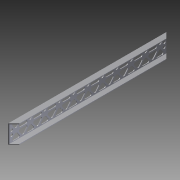
# Autodesk Inventor part: big U channel 3.25in
Saved by Autodesk Inventor 2012 (Build 160160000, 160)
## iProperties
Created: 2013-07-06
Part Number: big U channel 3.25in
Material: Default
Document SubType Name: Modeling
Designer: Bryce
Density: 1 g/cm^3
Author: Bryce
Autodesk Inventor part; units mm, degrees
ref_plane "YZ Plane" through (0, 0, 0) normal (1, 0, 0) x (0, 1, 0)
ref_plane "XZ Plane" through (0, 0, 0) normal (0, 1, 0) x (-1, 0, 0)
ref_plane "XY Plane" through (0, 0, 0) normal (0, 0, 1) x (1, 0, 0)
sketch "Sketch1" plane through (0, 0, 0) normal (0, 0, 1) x (1, 0, 0)
  line L0 (0, 0) -> (25.4, 0)
  line L1 (25.4, 82.55) -> (0, 82.55)
  line L2 (0, 82.55) -> (0, 0)
  line L3 (25.4, 79.375) -> (3.175, 79.375)
  line L4 (3.175, 79.375) -> (3.175, 3.175)
  line L5 (3.175, 3.175) -> (25.4, 3.175)
  line L6 (25.4, 82.55) -> (25.4, 79.375)
  line L7 (25.4, 3.175) -> (25.4, 0)
  dimension "d0" = 82.55
  dimension "d1" = 25.4
  dimension "d2" = 25.4
  dimension "d3" = 3.175
  dimension "d4" = 3.175
  dimension "d5" = 3.175
  constraints: 16 end point, 3 equal length, 3 perpendicular, 2 horizontal
  measures "d0" distance of L1.end L0.start
  measures "d1" distance of L1.start L1.end
  measures "d2" distance of L0.start L0.end
  measures "d3" distance between parallel lines of L1 L3
  measures "d4" distance between parallel lines of L2 L4
  measures "d5" distance between parallel lines of L0 L5
extrude "Extrusion1" add sketch "Sketch1" along normal blind 711.2
sketch "Sketch2" plane through (0, 82.55, 0) normal (0, 1, 0) x (1, 0, 0)
  line L0 (0, -711.2) -> (25.4, -711.2) projected
  line L1 (25.4, 0) -> (25.4, -711.2) projected
  line L2 (25.4, 0) -> (0, 0) projected
  line L3 (0, -711.2) -> (25.4, -685.8)
  line L4 (0, 0) -> (25.4, -25.4)
  dimension "d8" = 45
  constraints: 4 end point, 2 point on line, 1 perpendicular
  measures "d8" angle of L0 L3
extrude "Extrusion2" cut sketch "Sketch2" against normal through all
sketch "Sketch3" plane through (0, 0, 711.2) normal (-1, 0, 0) x (0, 0, 1)
  line L0 (0, 0) -> (0, 82.55) projected
  line L1 (-711.2, 82.55) -> (0, 82.55) projected
  line L2 (-711.2, 82.55) -> (-711.2, 0) projected
  line L3 (-711.2, 0) -> (0, 0) projected
  line L4 (-711.2, 41.275) -> (0, 41.275) construction
  line L5 (-711.2, 0) -> (-646.5455, 82.55) construction
  line L6 (-646.5455, 82.55) -> (-581.8909, 0) construction
  line L7 (-581.8909, 0) -> (-517.2364, 82.55) construction
  line L8 (-517.2364, 82.55) -> (-452.5818, 0) construction
  line L9 (-452.5818, 0) -> (-387.9273, 82.55) construction
  line L10 (-387.9273, 82.55) -> (-323.2727, 0) construction
  line L11 (-323.2727, 0) -> (-258.6182, 82.55) construction
  line L12 (-258.6182, 82.55) -> (-193.9636, 0) construction
  line L13 (-193.9636, 0) -> (-129.3091, 82.55) construction
  line L14 (-129.3091, 82.55) -> (-64.6545, 0) construction
  line L15 (-64.6545, 0) -> (0, 82.55) construction
  line L16 (-711.2, 82.55) -> (-646.5455, 0) construction
  line L17 (-646.5455, 0) -> (-581.8909, 82.55) construction
  line L18 (-581.8909, 82.55) -> (-517.2364, 0) construction
  line L19 (-517.2364, 0) -> (-452.5818, 82.55) construction
  line L20 (-452.5818, 82.55) -> (-387.9273, 0) construction
  line L21 (-387.9273, 0) -> (-323.2727, 82.55) construction
  line L22 (-323.2727, 82.55) -> (-258.6182, 0) construction
  line L23 (-258.6182, 0) -> (-193.9636, 82.55) construction
  line L24 (-193.9636, 82.55) -> (-129.3091, 0) construction
  line L25 (-129.3091, 0) -> (-64.6545, 82.55) construction
  line L26 (-64.6545, 82.55) -> (0, 0) construction
  line L27 (-702.1937, 6.35) -> (-678.8727, 36.1258)
  line L28 (-678.8727, 36.1258) -> (-655.5518, 6.35)
  line L29 (-655.5518, 6.35) -> (-702.1937, 6.35)
  line L30 (-672.3531, 38.1) -> (-646.5455, 5.1492)
  line L31 (-646.5455, 5.1492) -> (-620.7378, 38.1)
  line L32 (-620.7378, 38.1) -> (-672.3531, 38.1)
  line L33 (-704.85, 13.2568) -> (-685.3924, 38.1)
  line L34 (-685.3924, 38.1) -> (-704.85, 38.1)
  line L35 (-704.85, 38.1) -> (-704.85, 13.2568)
  line L36 (-704.85, 69.2932) -> (-704.85, 44.45)
  line L37 (-704.85, 44.45) -> (-685.3924, 44.45)
  line L38 (-685.3924, 44.45) -> (-704.85, 69.2932)
  line L39 (-702.1937, 76.2) -> (-678.8727, 46.4242)
  line L40 (-678.8727, 46.4242) -> (-655.5518, 76.2)
  line L41 (-655.5518, 76.2) -> (-702.1937, 76.2)
  line L42 (-672.3531, 44.45) -> (-646.5455, 77.4008)
  line L43 (-646.5455, 77.4008) -> (-620.7378, 44.45)
  line L44 (-620.7378, 44.45) -> (-672.3531, 44.45)
  line L45 (-637.5391, 6.35) -> (-614.2182, 36.1258)
  line L46 (-614.2182, 36.1258) -> (-590.8972, 6.35)
  line L47 (-590.8972, 6.35) -> (-637.5391, 6.35)
  line L48 (-607.6986, 38.1) -> (-581.8909, 5.1492)
  line L49 (-581.8909, 5.1492) -> (-556.0833, 38.1)
  line L50 (-556.0833, 38.1) -> (-607.6986, 38.1)
  line L51 (-637.5391, 76.2) -> (-614.2182, 46.4242)
  line L52 (-614.2182, 46.4242) -> (-590.8972, 76.2)
  line L53 (-590.8972, 76.2) -> (-637.5391, 76.2)
  line L54 (-607.6986, 44.45) -> (-581.8909, 77.4008)
  line L55 (-581.8909, 77.4008) -> (-556.0833, 44.45)
  line L56 (-556.0833, 44.45) -> (-607.6986, 44.45)
  line L57 (-572.8846, 6.35) -> (-549.5636, 36.1258)
  line L58 (-549.5636, 36.1258) -> (-526.2427, 6.35)
  line L59 (-526.2427, 6.35) -> (-572.8846, 6.35)
  line L60 (-543.044, 38.1) -> (-517.2364, 5.1492)
  line L61 (-517.2364, 5.1492) -> (-491.4287, 38.1)
  line L62 (-491.4287, 38.1) -> (-543.044, 38.1)
  line L63 (-572.8846, 76.2) -> (-549.5636, 46.4242)
  line L64 (-549.5636, 46.4242) -> (-526.2427, 76.2)
  line L65 (-526.2427, 76.2) -> (-572.8846, 76.2)
  line L66 (-543.044, 44.45) -> (-517.2364, 77.4008)
  line L67 (-517.2364, 77.4008) -> (-491.4287, 44.45)
  line L68 (-491.4287, 44.45) -> (-543.044, 44.45)
  line L69 (-508.23, 6.35) -> (-484.9091, 36.1258)
  line L70 (-484.9091, 36.1258) -> (-461.5882, 6.35)
  line L71 (-461.5882, 6.35) -> (-508.23, 6.35)
  line L72 (-478.3895, 38.1) -> (-452.5818, 5.1492)
  line L73 (-452.5818, 5.1492) -> (-426.7742, 38.1)
  line L74 (-426.7742, 38.1) -> (-478.3895, 38.1)
  line L75 (-508.23, 76.2) -> (-484.9091, 46.4242)
  line L76 (-484.9091, 46.4242) -> (-461.5882, 76.2)
  line L77 (-461.5882, 76.2) -> (-508.23, 76.2)
  line L78 (-478.3895, 44.45) -> (-452.5818, 77.4008)
  line L79 (-452.5818, 77.4008) -> (-426.7742, 44.45)
  line L80 (-426.7742, 44.45) -> (-478.3895, 44.45)
  line L81 (-443.5755, 6.35) -> (-420.2545, 36.1258)
  line L82 (-420.2545, 36.1258) -> (-396.9336, 6.35)
  line L83 (-396.9336, 6.35) -> (-443.5755, 6.35)
  line L84 (-413.7349, 38.1) -> (-387.9273, 5.1492)
  line L85 (-387.9273, 5.1492) -> (-362.1196, 38.1)
  line L86 (-362.1196, 38.1) -> (-413.7349, 38.1)
  line L87 (-443.5755, 76.2) -> (-420.2545, 46.4242)
  line L88 (-420.2545, 46.4242) -> (-396.9336, 76.2)
  line L89 (-396.9336, 76.2) -> (-443.5755, 76.2)
  line L90 (-413.7349, 44.45) -> (-387.9273, 77.4008)
  line L91 (-387.9273, 77.4008) -> (-362.1196, 44.45)
  line L92 (-362.1196, 44.45) -> (-413.7349, 44.45)
  line L93 (-378.9209, 6.35) -> (-355.6, 36.1258)
  line L94 (-355.6, 36.1258) -> (-332.2791, 6.35)
  line L95 (-332.2791, 6.35) -> (-378.9209, 6.35)
  line L96 (-349.0804, 38.1) -> (-323.2727, 5.1492)
  line L97 (-323.2727, 5.1492) -> (-297.4651, 38.1)
  line L98 (-297.4651, 38.1) -> (-349.0804, 38.1)
  line L99 (-378.9209, 76.2) -> (-355.6, 46.4242)
  line L100 (-355.6, 46.4242) -> (-332.2791, 76.2)
  line L101 (-332.2791, 76.2) -> (-378.9209, 76.2)
  line L102 (-349.0804, 44.45) -> (-323.2727, 77.4008)
  line L103 (-323.2727, 77.4008) -> (-297.4651, 44.45)
  line L104 (-297.4651, 44.45) -> (-349.0804, 44.45)
  line L105 (-314.2664, 6.35) -> (-290.9455, 36.1258)
  line L106 (-290.9455, 36.1258) -> (-267.6245, 6.35)
  line L107 (-267.6245, 6.35) -> (-314.2664, 6.35)
  line L108 (-284.4258, 38.1) -> (-258.6182, 5.1492)
  line L109 (-258.6182, 5.1492) -> (-232.8105, 38.1)
  line L110 (-232.8105, 38.1) -> (-284.4258, 38.1)
  line L111 (-314.2664, 76.2) -> (-290.9455, 46.4242)
  line L112 (-290.9455, 46.4242) -> (-267.6245, 76.2)
  line L113 (-267.6245, 76.2) -> (-314.2664, 76.2)
  line L114 (-284.4258, 44.45) -> (-258.6182, 77.4008)
  line L115 (-258.6182, 77.4008) -> (-232.8105, 44.45)
  line L116 (-232.8105, 44.45) -> (-284.4258, 44.45)
  line L117 (-249.6118, 6.35) -> (-226.2909, 36.1258)
  line L118 (-226.2909, 36.1258) -> (-202.97, 6.35)
  line L119 (-202.97, 6.35) -> (-249.6118, 6.35)
  line L120 (-219.7713, 38.1) -> (-193.9636, 5.1492)
  line L121 (-193.9636, 5.1492) -> (-168.156, 38.1)
  line L122 (-168.156, 38.1) -> (-219.7713, 38.1)
  line L123 (-249.6118, 76.2) -> (-226.2909, 46.4242)
  line L124 (-226.2909, 46.4242) -> (-202.97, 76.2)
  line L125 (-202.97, 76.2) -> (-249.6118, 76.2)
  line L126 (-219.7713, 44.45) -> (-193.9636, 77.4008)
  line L127 (-193.9636, 77.4008) -> (-168.156, 44.45)
  line L128 (-168.156, 44.45) -> (-219.7713, 44.45)
  line L129 (-184.9573, 6.35) -> (-161.6364, 36.1258)
  line L130 (-161.6364, 36.1258) -> (-138.3154, 6.35)
  line L131 (-138.3154, 6.35) -> (-184.9573, 6.35)
  line L132 (-155.1167, 38.1) -> (-129.3091, 5.1492)
  line L133 (-129.3091, 5.1492) -> (-103.5014, 38.1)
  line L134 (-103.5014, 38.1) -> (-155.1167, 38.1)
  line L135 (-184.9573, 76.2) -> (-161.6364, 46.4242)
  line L136 (-161.6364, 46.4242) -> (-138.3154, 76.2)
  line L137 (-138.3154, 76.2) -> (-184.9573, 76.2)
  line L138 (-155.1167, 44.45) -> (-129.3091, 77.4008)
  line L139 (-129.3091, 77.4008) -> (-103.5014, 44.45)
  line L140 (-103.5014, 44.45) -> (-155.1167, 44.45)
  line L141 (-120.3028, 6.35) -> (-96.9818, 36.1258)
  line L142 (-96.9818, 36.1258) -> (-73.6609, 6.35)
  line L143 (-73.6609, 6.35) -> (-120.3028, 6.35)
  line L144 (-90.4622, 38.1) -> (-64.6545, 5.1492)
  line L145 (-64.6545, 5.1492) -> (-38.8469, 38.1)
  line L146 (-38.8469, 38.1) -> (-90.4622, 38.1)
  line L147 (-120.3028, 76.2) -> (-96.9818, 46.4242)
  line L148 (-96.9818, 46.4242) -> (-73.6609, 76.2)
  line L149 (-73.6609, 76.2) -> (-120.3028, 76.2)
  line L150 (-90.4622, 44.45) -> (-64.6545, 77.4008)
  line L151 (-64.6545, 77.4008) -> (-38.8469, 44.45)
  line L152 (-38.8469, 44.45) -> (-90.4622, 44.45)
  line L153 (-55.6482, 6.35) -> (-32.3273, 36.1258)
  line L154 (-32.3273, 36.1258) -> (-9.0063, 6.35)
  line L155 (-9.0063, 6.35) -> (-55.6482, 6.35)
  line L156 (-32.3273, 46.4242) -> (-55.6482, 76.2)
  line L157 (-55.6482, 76.2) -> (-9.0063, 76.2)
  line L158 (-9.0063, 76.2) -> (-32.3273, 46.4242)
  line L159 (-6.35, 69.2932) -> (-25.8076, 44.45)
  line L160 (-25.8076, 44.45) -> (-6.35, 44.45)
  line L161 (-6.35, 44.45) -> (-6.35, 69.2932)
  line L162 (-25.8076, 38.1) -> (-6.35, 13.2568)
  line L163 (-6.35, 13.2568) -> (-6.35, 38.1)
  line L164 (-6.35, 38.1) -> (-25.8076, 38.1)
  point P0 (-637.5391, 6.35)
  dimension "d11" = 76.137
  dimension "d12" = 38.069
  dimension "d13" = 6.35
  dimension "d14" = 3.175
  dimension "d15" = 3.175
  dimension "d16" = 3.175
  dimension "d17" = 3.175
  dimension "d18" = 6.35
  dimension "d19" = 3.175
  dimension "d20" = 3.175
  dimension "d21" = 6.35
  dimension "d22" = 3.175
  dimension "d23" = 3.175
  dimension "d24" = 6.35
  dimension "d25" = 3.175
  dimension "d26" = 3.175
  dimension "d27" = 3.175
  dimension "d28" = 3.175
  dimension "d29" = 3.175
  dimension "d30" = 3.175
  dimension "d31" = 3.175
  dimension "d32" = 6.35
  dimension "d34" = 64.6546
  dimension "d37" = 64.6546
  dimension "d42" = 3.175
  dimension "d43" = 3.175
  dimension "d44" = 3.175
  dimension "d45" = 3.175
  dimension "d46" = 6.35
  dimension "d47" = 3.175
  dimension "d48" = 3.175
  dimension "d49" = 6.35
  dimension "d50" = 3.175
  dimension "d51" = 6.35
  dimension "d52" = 3.175
  dimension "d53" = 6.35
  constraints: 322 end point, 116 parallel, 108 horizontal alignment, 37 collinear, 2 midpoint, 2 perpendicular, 1 horizontal, 22 other
  measures "d11" angle of L6 L5
  measures "d12" angle of L2 L5
  measures "d13" distance of the line from the sketch origin of L29
  measures "d14" distance between parallel lines of L5 L27
  measures "d15" distance between parallel lines of L16 L28
  measures "d16" distance between parallel lines of L5 L33
  measures "d17" distance between parallel lines of L4 L34
  measures "d18" distance between parallel lines of L2 L35
  measures "d19" distance between parallel lines of L4 L37
  measures "d20" distance between parallel lines of L16 L38
  measures "d21" distance between parallel lines of L2 L36
  measures "d22" distance between parallel lines of L39 L16
  measures "d23" distance between parallel lines of L5 L40
  measures "d25" distance between parallel lines of L5 L42
  measures "d26" distance between parallel lines of L4 L44
  measures "d27" distance between parallel lines of L16 L30
  measures "d28" distance between parallel lines of L4 L32
  measures "d29" distance between parallel lines of L17 L31
  measures "d30" distance between parallel lines of L6 L43
  measures "d31" distance from line of L17 point (-637.539, 6.35)
  measures "d34" distance of point (-637.539, 6.35) L27.start
  measures "d37" distance of L27.start L45.start
  measures "d42" distance between parallel lines of L15 L153
  measures "d43" distance between parallel lines of L26 L154
  measures "d44" distance between parallel lines of L162 L26
  measures "d45" distance between parallel lines of L4 L164
  measures "d46" distance between parallel lines of L0 L163
  measures "d47" distance between parallel lines of L4 L160
  measures "d48" distance between parallel lines of L15 L159
  measures "d49" distance between parallel lines of L0 L161
  measures "d50" distance between parallel lines of L15 L158
  measures "d51" distance of the line from the sketch origin of L155
  measures "d52" distance between parallel lines of L26 L156
extrude "Extrusion3" cut sketch "Sketch3" against normal through all contours L27 L28 L29 | L32 L31 L30 | L35 L34 L33 | L38 L37 L36 | L41 L40 L39 | L42 L43 L44 | L45 L46 L47 | L50 L49 L48 | L53 L52 L51 | L54 L55 L56 | L57 L58 L59 | L62 L61 L60 | L65 L64 L63 | L66 L67 L68 | L69 L70 L71 | L74 L73 L72 | L77 L76 L75 | L78 L79 L80 | L81 L82 L83 | L86 L85 L84 | L89 L88 L87 | L90 L91 L92 | L93 L94 L95 | L98 L97 L96 | L101 L100 L99 | L102 L103 L104 | L105 L106 L107 | L110 L109 L108 | L113 L112 L111 | L114 L115 L116 | L117 L118 L119 | L122 L121 L120 | L125 L124 L123 | L126 L127 L128 | L129 L130 L131 | L134 L133 L132 | L137 L136 L135 | L138 L139 L140 | L141 L142 L143 | L146 L145 L144 | L149 L148 L147 | L150 L151 L152 | L153 L154 L155 | L156 L157 L158 | L161 L160 L159 | L164 L163 L162
fillet "Fillet1" radius 6.35 136 edges at (1.5875, 6.35, 9.0063) (1.5875, 13.2568, 6.35) (1.5875, 38.1, 6.35) (1.5875, 38.1, 25.8076) (1.5875, 69.2932, 6.35) (1.5875, 44.45, 6.35) (1.5875, 44.45, 25.8076) (1.5875, 76.2, 55.6482) (1.5875, 76.2, 9.0063) (1.5875, 46.4242, 32.3273) (1.5875, 44.45, 38.8469) (1.5875, 36.1258, 32.3273) (1.5875, 38.1, 38.8469) (1.5875, 6.35, 55.6482) (1.5875, 5.1492, 64.6545) (1.5875, 38.1, 90.4622) (1.5875, 44.45, 90.4622) (1.5875, 77.4008, 64.6545) (1.5875, 76.2, 120.3028) (1.5875, 76.2, 73.6609) (1.5875, 46.4242, 96.9818) (1.5875, 44.45, 103.5014) (1.5875, 77.4008, 129.3091) (1.5875, 44.45, 155.1167) (1.5875, 38.1, 103.5014) (1.5875, 36.1258, 96.9818) (1.5875, 6.35, 73.6609) (1.5875, 6.35, 120.3028) (1.5875, 6.35, 138.3154) (1.5875, 5.1492, 129.3091) (1.5875, 38.1, 155.1167) (1.5875, 46.4242, 161.6364) (1.5875, 36.1258, 161.6364) (1.5875, 77.4008, 193.9636) (1.5875, 44.45, 168.156) (1.5875, 44.45, 219.7713) (1.5875, 38.1, 168.156) (1.5875, 6.35, 184.9573) (1.5875, 5.1492, 193.9636) (1.5875, 38.1, 219.7713) (1.5875, 44.45, 232.8105) (1.5875, 46.4242, 226.2909) (1.5875, 76.2, 249.6118) (1.5875, 77.4008, 258.6182) (1.5875, 76.2, 267.6245) (1.5875, 44.45, 284.4258) (1.5875, 38.1, 232.8105) (1.5875, 36.1258, 226.2909) (1.5875, 6.35, 249.6118) (1.5875, 6.35, 267.6245) (1.5875, 6.35, 202.97) (1.5875, 5.1492, 258.6182) (1.5875, 6.35, 314.2664) (1.5875, 76.2, 314.2664) (1.5875, 46.4242, 290.9455) (1.5875, 38.1, 284.4258) (1.5875, 44.45, 297.4651) (1.5875, 38.1, 297.4651) (1.5875, 44.45, 349.0804) (1.5875, 77.4008, 323.2727) (1.5875, 46.4242, 355.6) (1.5875, 38.1, 349.0804) (1.5875, 5.1492, 323.2727) (1.5875, 6.35, 332.2791) (1.5875, 36.1258, 355.6) (1.5875, 76.2, 332.2791) (1.5875, 76.2, 378.9209) (1.5875, 76.2, 138.3154) (1.5875, 76.2, 184.9573) (1.5875, 38.1, 362.1196) (1.5875, 36.1258, 290.9455) (1.5875, 6.35, 378.9209) (1.5875, 5.1492, 387.9273) (1.5875, 44.45, 362.1196) (1.5875, 77.4008, 387.9273) (1.5875, 44.45, 413.7349) (1.5875, 36.1258, 420.2545) (1.5875, 44.45, 426.7742) (1.5875, 46.4242, 420.2545) (1.5875, 38.1, 413.7349) (1.5875, 76.2, 396.9336) (1.5875, 76.2, 443.5755) (1.5875, 6.35, 396.9336) (1.5875, 38.1, 426.7742) (1.5875, 5.1492, 452.5818) (1.5875, 38.1, 478.3895) (1.5875, 44.45, 478.3895) (1.5875, 77.4008, 452.5818) (1.5875, 76.2, 461.5882) (1.5875, 46.4242, 484.9091) (1.5875, 76.2, 508.23) (1.5875, 6.35, 461.5882) (1.5875, 36.1258, 484.9091) (1.5875, 6.35, 508.23) (1.5875, 44.45, 491.4287) (1.5875, 38.1, 491.4287) (1.5875, 5.1492, 517.2364) (1.5875, 6.35, 526.2427) (1.5875, 77.4008, 517.2364) (1.5875, 38.1, 543.044) (1.5875, 44.45, 543.044) (1.5875, 76.2, 526.2427) (1.5875, 36.1258, 549.5636) (1.5875, 46.4242, 549.5636) (1.5875, 76.2, 572.8846) (1.5875, 6.35, 572.8846) (1.5875, 38.1, 556.0833) (1.5875, 44.45, 556.0833) (1.5875, 5.1492, 581.8909) (1.5875, 38.1, 607.6986) (1.5875, 44.45, 607.6986) (1.5875, 77.4008, 581.8909) (1.5875, 6.35, 590.8972) (1.5875, 76.2, 590.8972) (1.5875, 76.2, 637.5391) (1.5875, 36.1258, 614.2182) (1.5875, 46.4242, 614.2182) (1.5875, 6.35, 637.5391) (1.5875, 38.1, 620.7378) (1.5875, 44.45, 620.7378) (1.5875, 77.4008, 646.5455) (1.5875, 44.45, 672.3531) (1.5875, 5.1492, 646.5455) (1.5875, 38.1, 672.3531) (1.5875, 36.1258, 678.8727) (1.5875, 46.4242, 678.8727) (1.5875, 6.35, 655.5518) (1.5875, 76.2, 655.5518) (1.5875, 76.2, 702.1937) (1.5875, 69.2932, 704.85) (1.5875, 44.45, 704.85) (1.5875, 44.45, 685.3924) (1.5875, 38.1, 685.3924) (1.5875, 38.1, 704.85) (1.5875, 13.2568, 704.85) (1.5875, 6.35, 702.1937)
equation "\"d4\" = d3"
equation "\"d5\" = d4"
equation "\"d11\" = 2 * d12"
equation "\"d15\" = d14"
equation "\"d16\" = d14"
equation "\"d17\" = d16"
equation "\"d18\" = d13"
equation "\"d19\" = d17"
equation "\"d20\" = d19"
equation "\"d21\" = d18"
equation "\"d22\" = d20"
equation "\"d23\" = d20"
equation "\"d24\" = d21"
equation "\"d25\" = d23"
equation "\"d26\" = d25"
equation "\"d27\" = d15"
equation "\"d28\" = d26"
equation "\"d29\" = d27"
equation "\"d30\" = d26"
equation "\"d31\" = d27"
equation "\"d32\" = d13"
equation "\"d37\" = d34"
equation "\"d42\" = d14"
equation "\"d43\" = d42"
equation "\"d44\" = d42"
equation "\"d45\" = d42"
equation "\"d46\" = d51"
equation "\"d47\" = d42"
equation "\"d48\" = d42"
equation "\"d49\" = d46"
equation "\"d50\" = d42"
equation "\"d51\" = d13"
equation "\"d52\" = d42"
equation "\"d53\" = d49"
body "Solid1"
